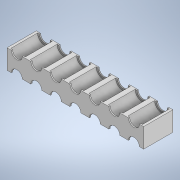
# Autodesk Inventor part: mid_insert
Saved by Autodesk Inventor 2021 (Build 250183000, 183)
## iProperties
Created: 2021-06-03
Part Number: mid_insert
Material: Generic
Document SubType Name: Modeling
Designer: Anton
Density: 1 g/cm^3
Appearance: Default
Author: Anton
Autodesk Inventor part; units mm, degrees
ref_plane "YZ Plane" through (0, 0, 0) normal (1, 0, 0) x (0, 1, 0)
ref_plane "XZ Plane" through (0, 0, 0) normal (0, 1, 0) x (-1, 0, 0)
ref_plane "XY Plane" through (0, 0, 0) normal (0, 0, 1) x (1, 0, 0)
sketch "Sketch1" plane through (0, 0, 0) normal (0, 0, 1) x (1, 0, 0)
  arc A0 (-3, 0) -> (3, 0) centre (0, 0) ccw
  line L0 (-3, 0) -> (-5.517, 0)
  line L1 (3, 0) -> (5.517, 0)
  line L2 (4, 0) -> (4, -8)
  line L3 (-4, -8) -> (-4, 0)
  line L4 (-4, 0) -> (-3, 0)
  line L5 (3, 0) -> (4, 0)
  arc A1 (3, -8) -> (-3, -8) centre (0, -8) ccw
  line L6 (4, -8) -> (3, -8)
  line L7 (-3, -8) -> (-4, -8)
  dimension "d0" = 6
  dimension "d1" = 1
  dimension "d2" = 1
  dimension "d4" = 6
  dimension "d5" = 8
  dimension "d6" = 8
  dimension "d7" = 8
  constraints: 16 end point, 5 parallel, 4 horizontal, 4 point on circle, 2 centre point, 2 perpendicular, 1 coincident, 1 point on line
  measures "d0" diameter of A0
  measures "d1" distance from line of L0.start L3
  measures "d2" distance from line of L2 L1.start
  measures "d4" diameter of A1
  measures "d5" distance between parallel lines of L2 L3
  measures "d6" distance between parallel lines of L1 L6
  measures "d7" distance between parallel lines of L0 L7
extrude "Extrusion1" add sketch "Sketch1" along normal blind 11
pattern_linear "Rectangular Pattern1" count 7 spacing 8 along (-1, 0, 0) of "Extrusion1"
sketch "Sketch2" plane through (0, 0, 0) normal (0, 0, -1) x (-1, 0, 0)
  line L0 (-4, -8) -> (-4, 0) projected
  line L1 (52, 0) -> (52, -8) projected
  line L2 (-4, 0) -> (52, 0)
  line L3 (52, 0) -> (52, -8)
  line L4 (52, -8) -> (-4, -8)
  line L5 (-4, -8) -> (-4, 0)
  point P0 (0, 0)
  constraints: 8 end point, 2 parallel, 1 horizontal, 1 perpendicular
extrude "Extrusion2" add sketch "Sketch2" along normal blind 0.5
sketch "Sketch3" plane through (0, 0, 11) normal (0, 0, 1) x (1, 0, 0)
  line L0 (4, 0) -> (3, 0) projected
  line L1 (4, -8) -> (-52, -8) projected
  line L2 (4, 0) -> (-52, 0)
  line L3 (-52, 0) -> (-52, -8)
  line L4 (-52, -8) -> (4, -8)
  line L5 (4, -8) -> (4, 0)
  point P0 (0, 0)
  constraints: 8 end point, 2 parallel, 1 horizontal, 1 perpendicular
extrude "Extrusion3" add sketch "Sketch3" along normal blind 0.5
sketch "Sketch4" plane through (0, 0, 11.5) normal (0, 0, 1) x (1, 0, 0)
  line L0 (-52, 0) -> (4, 0) projected
  circle A0 centre (-48, 0) radius 2.25
  line L1 (4, -8) -> (-52, -8) projected
  circle A1 centre (-48, -8) radius 2.25
  line L2 (-52, 0) -> (-52, -8) projected
  circle A2 centre (-40, 0) radius 2.25
  circle A3 centre (-40, -8) radius 2.25
  circle A4 centre (-32, 0) radius 2.25
  circle A5 centre (-32, -8) radius 2.25
  circle A6 centre (-24, 0) radius 2.25
  circle A7 centre (-24, -8) radius 2.25
  circle A8 centre (-16, 0) radius 2.25
  circle A9 centre (-16, -8) radius 2.25
  circle A10 centre (-8, 0) radius 2.25
  circle A11 centre (-8, -8) radius 2.25
  circle A12 centre (0, 0) radius 2.25
  circle A13 centre (0, -8) radius 2.25
  point P0 (0, 0)
  point P1 (-50.25, -8)
  point P2 (-45.75, -8)
  point P3 (-42.25, -8)
  point P4 (-37.75, -8)
  point P5 (-34.25, -8)
  point P6 (-29.75, -8)
  point P7 (-26.25, -8)
  point P8 (-21.75, -8)
  point P9 (-18.25, -8)
  point P10 (-13.75, -8)
  point P11 (-10.25, -8)
  point P12 (-5.75, -8)
  point P13 (-5.75, 0)
  point P14 (-10.25, 0)
  point P15 (-13.75, 0)
  point P16 (-18.25, 0)
  point P17 (-21.75, 0)
  point P18 (-26.25, 0)
  point P19 (-29.75, 0)
  point P20 (-34.25, 0)
  point P21 (-37.75, 0)
  point P22 (-42.25, 0)
  point P23 (-45.75, 0)
  point P24 (-50.25, 0)
  point P25 (-2.25, -8)
  point P26 (2.25, -8)
  point P27 (2.25, 0)
  point P28 (-2.25, 0)
  dimension "d17" = 4.5
  dimension "d18" = 4.5
  dimension "d19" = 4
  dimension "d20" = 4
  dimension "d23" = 8
  constraints: 14 centre point, 2 point on line, 1 horizontal, 24 other
  measures "d17" diameter of A0
  measures "d18" diameter of A1
  measures "d19" distance of L0.start A0.centre
  measures "d20" distance from line of L2 A1.centre
  measures "d23" distance of A0.centre A2.centre
extrude "Extrusion4" cut sketch "Sketch4" along normal blind 50 and the other way blind 20 contours L0 A0 | L0 A2 | L0 A4 | L0 A6 | L0 A8 | L0 A10 | L0 A12 | L1 A13 | L1 A11 | L1 A9 | L1 A7 | L1 A5 | L1 A3 | L1 A1 picked at (-48.0904, -0.7445) picked at (-40.0904, -0.7445) picked at (-32.0904, -0.7445) picked at (-24.0904, -0.7445) picked at (-16.6641, -0.3485) picked at (-8.5396, -0.6768) picked at (-0.0904, -0.7445) picked at (0.426, -7.3828) picked at (-8.6859, -7.472) picked at (-15.4386, -7.5027) picked at (-23.9096, -7.2555) picked at (-31.9096, -7.2555) picked at (-39.4386, -7.5027) picked at (-47.4386, -7.5027)
body "Solid1"
